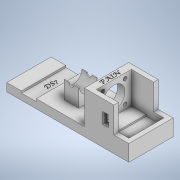
# Autodesk Inventor part: GN_StepperMount_v3
Saved by Autodesk Inventor 2020 (Build 240168000, 168)
## iProperties
Created: 2021-12-03
Part Number: GN_StepperMount_v3
Material: Generic
Document SubType Name: Modeling
Designer: bi19884
Density: 1 g/cm^3
Appearance: Default
Author: bi19884
Autodesk Inventor part; units mm, degrees
ref_plane "YZ Plane" through (0, 0, 0) normal (1, 0, 0) x (0, 1, 0)
ref_plane "XZ Plane" through (0, 0, 0) normal (0, 1, 0) x (-1, 0, 0)
ref_plane "XY Plane" through (0, 0, 0) normal (0, 0, 1) x (1, 0, 0)
sketch "Sketch1" plane through (0, 0, 0) normal (0, 1, 0) x (-1, 0, 0)
  line L0 (10.1329, 50.4274) -> (-115.1171, 50.4274)
  line L1 (-115.1171, 50.4274) -> (-115.1171, -9.5726)
  line L2 (-115.1171, -9.5726) -> (10.1329, -9.5726)
  line L3 (10.1329, -9.5726) -> (10.1329, 50.4274)
  point P0 (0, 0)
  dimension "d0" = 125.25
  dimension "d1" = 60
  constraints: 8 end point, 2 parallel, 1 horizontal, 1 perpendicular
  measures "d0" distance of L1.end L2.end
  measures "d1" distance of L2.end L0.start
extrude "Extrusion1" add sketch "Sketch1" along normal blind 12
sketch "Sketch2" plane through (-10.1329, 0, -9.5726) normal (-1, 0, 0) x (0, 0, 1)
  line L0 (0, 8.5) -> (60, 8.5)
  line L1 (60, 8.5) -> (60, 0)
  line L2 (60, 0) -> (0, 0)
  line L3 (0, 0) -> (0, 8.5)
  line L4 (0, 0) -> (0, 12) projected
  line L5 (0, 0) -> (60, 0) projected
  point P0 (9.5726, 0)
  dimension "d4" = 8.5
  dimension "d5" = 60
  dimension "d6" = 0
  dimension "d7" = 0
  constraints: 8 end point, 2 parallel, 1 horizontal, 1 perpendicular
  measures "d4" distance between parallel lines of L0 L2
  measures "d5" distance between parallel lines of L1 L3
  measures "d6" distance between parallel lines of L4 L3
  measures "d7" distance between parallel lines of L5 L2
extrude "Extrusion2" add sketch "Sketch2" along normal blind 40
sketch "Sketch4" plane through (0, 12, 0) normal (0, 1, 0) x (1, 0, 0)
  line L0 (115.1171, 9.5726) -> (-10.1329, 9.5726) projected
  line L1 (-10.1329, -50.4274) -> (115.1171, -50.4274) projected
  line L2 (115.1171, -50.4274) -> (115.1171, 9.5726) projected
  line L3 (-10.1329, 9.5726) -> (-10.1329, -50.4274) projected
  line L4 (9.8671, -7.9274) -> (29.8671, -7.9274)
  line L5 (29.8671, -7.9274) -> (29.8671, -32.9274)
  line L6 (29.8671, -32.9274) -> (9.8671, -32.9274)
  line L7 (9.8671, -32.9274) -> (9.8671, -7.9274)
  point P0 (0, 0)
  dimension "d15" = 60
  dimension "d16" = 125.25
  dimension "d17" = 25
  dimension "d18" = 20
  dimension "d19" = 17.5
  dimension "d20" = 17.5
  dimension "d21" = 20
  constraints: 8 end point, 2 parallel, 1 horizontal, 1 perpendicular
  measures "d15" distance between parallel lines of L0 L1
  measures "d16" distance between parallel lines of L2 L3
  measures "d17" distance between parallel lines of L4 L6
  measures "d18" distance between parallel lines of L5 L7
  measures "d19" distance between parallel lines of L1 L6
  measures "d20" distance between parallel lines of L0 L4
  measures "d21" distance between parallel lines of L3 L7
extrude "Extrusion3" add sketch "Sketch4" along normal blind 23.5 contours L4 L5 L6 L7
sketch "Sketch6" plane through (29.8671, 12, 32.9274) normal (1, 0, 0) x (0, 0, -1)
  circle A0 centre (12.5, 23.5) radius 11.5
  line L0 (0, 23.5) -> (25, 23.5) projected
  line L1 (25, 0) -> (25, 23.5) projected
  line L2 (0, 0) -> (0, 23.5) projected
  line L3 (-17.5, 0) -> (42.5, 0) projected
  point P0 (32.9274, -12)
  point P1 (24, 23.5)
  point P2 (1, 23.5)
  dimension "d24" = 23
  dimension "d25" = 0
  dimension "d26" = 12.5
  dimension "d27" = 25
  dimension "d153" = 23.5
  constraints: 1 centre point
  measures "d24" diameter of A0
  measures "d25" distance from line of L0 A0.centre
  measures "d26" distance from line of L1 A0.centre
  measures "d27" distance between parallel lines of L2 L1
  measures "d153" distance from line of L3 A0.centre
extrude "Extrusion4" cut sketch "Sketch6" against normal blind 20 contours A0 L0 picked at (10.3224, 16.7824)
sketch "Sketch7" plane through (9.8671, 12, 32.9274) normal (0, 0, 1) x (1, 0, 0)
  circle A0 centre (10, 23.5) radius 3.5
  line L0 (0, 23.5) -> (20, 23.5) projected
  line L1 (0, 0) -> (0, 23.5) projected
  line L2 (20, 0) -> (20, 23.5) projected
  point P0 (-9.8671, -12)
  point P1 (13.5, 23.5)
  point P2 (6.5, 23.5)
  dimension "d30" = 7
  dimension "d31" = 0
  dimension "d32" = 20
  dimension "d33" = 10
  dimension "d34" = 10
  constraints: 1 centre point
  measures "d30" diameter of A0
  measures "d31" distance from line of L0 A0.centre
  measures "d32" distance between parallel lines of L1 L2
  measures "d33" distance from line of L2 A0.centre
  measures "d34" distance from line of L1 A0.centre
extrude "Extrusion5" cut sketch "Sketch7" against normal blind 25 contours A0 L0 picked at (11.1667, 22.4156)
sketch "Sketch8" plane through (0, 12, 0) normal (0, 1, 0) x (1, 0, 0)
  line L0 (64.8671, 9.5726) -> (54.8671, 9.5726)
  line L1 (54.8671, 9.5726) -> (54.8671, -50.4274)
  line L2 (54.8671, -50.4274) -> (64.8671, -50.4274)
  line L3 (64.8671, -50.4274) -> (64.8671, 9.5726)
  line L4 (-10.1329, 9.5726) -> (-10.1329, -50.4274) projected
  line L5 (-10.1329, -50.4274) -> (115.1171, -50.4274) projected
  line L6 (115.1171, 9.5726) -> (-10.1329, 9.5726) projected
  point P0 (0, 0)
  dimension "d37" = 65
  dimension "d38" = 10
  dimension "d39" = 0
  dimension "d40" = 60
  dimension "d41" = 60
  dimension "d42" = 0
  constraints: 8 end point, 2 parallel, 1 horizontal, 1 perpendicular
  measures "d37" distance between parallel lines of L4 L1
  measures "d38" distance between parallel lines of L1 L3
  measures "d39" distance between parallel lines of L5 L2
  measures "d40" distance of L0.end L1.end
  measures "d41" distance between parallel lines of L5 L6
  measures "d42" distance between parallel lines of L6 L0
extrude "Extrusion6" add sketch "Sketch8" along normal blind 45 contours L3 L2 L1 L0
sketch "Sketch9" plane through (0, 12, 0) normal (0, 1, 0) x (1, 0, 0)
  line L0 (108.8671, 9.5726) -> (115.1171, 9.5726)
  line L1 (115.1171, 9.5726) -> (115.1171, -50.4274)
  line L2 (115.1171, -50.4274) -> (108.8671, -50.4274)
  line L3 (108.8671, -50.4274) -> (108.8671, 9.5726)
  line L4 (64.8671, -50.4274) -> (64.8671, 9.5726) projected
  line L5 (54.8671, 9.5726) -> (54.8671, -50.4274) projected
  line L6 (29.8671, -8.9274) -> (29.8671, -31.9274) projected
  line L7 (115.1171, 9.5726) -> (-10.1329, 9.5726) projected
  line L8 (64.8671, 9.5726) -> (54.8671, 9.5726) projected
  line L9 (-10.1329, -50.4274) -> (115.1171, -50.4274) projected
  line L10 (54.8671, -50.4274) -> (64.8671, -50.4274) projected
  line L11 (115.1171, -50.4274) -> (115.1171, 9.5726) projected
  point P0 (0, 0)
  dimension "d45" = 6.25
  dimension "d46" = 44
  dimension "d47" = 25
  dimension "d48" = 0
  dimension "d49" = 60
  dimension "d50" = 0
  dimension "d51" = 0
  dimension "d52" = 60
  dimension "d69" = 0
  constraints: 8 end point, 2 parallel, 1 horizontal, 1 perpendicular
  measures "d45" distance between parallel lines of L1 L3
  measures "d46" distance between parallel lines of L4 L3
  measures "d47" distance between parallel lines of L5 L6
  measures "d48" distance between parallel lines of L7 L0
  measures "d49" distance between parallel lines of L2 L0
  measures "d50" distance between parallel lines of L7 L8
  measures "d51" distance from line of L9 L2.end
  measures "d52" distance between parallel lines of L10 L8
  measures "d69" distance between parallel lines of L11 L1
extrude "Extrusion7" add sketch "Sketch9" along normal blind 10 contours L0 L1 L2 L3
sketch "Sketch10" plane through (64.8671, 12, 50.4274) normal (1, 0, 0) x (0, 0, -1)
  circle A0 centre (30, 23.5) radius 15
  line L0 (0, 0) -> (0, 45) projected
  line L1 (60, 0) -> (60, 45) projected
  line L2 (0, 0) -> (60, 0) projected
  line L3 (0, 45) -> (60, 45) projected
  point P0 (50.4274, -12)
  dimension "d55" = 30
  dimension "d56" = 30
  dimension "d57" = 30
  dimension "d58" = 60
  dimension "d59" = 23.5
  dimension "d60" = 21.5
  constraints: 1 centre point
  measures "d55" diameter of A0
  measures "d56" distance from line of L0 A0.centre
  measures "d57" distance from line of L1 A0.centre
  measures "d58" distance between parallel lines of L1 L0
  measures "d59" distance from line of L2 A0.centre
  measures "d60" distance from line of L3 A0.centre
extrude "Extrusion8" cut sketch "Sketch10" against normal blind 10 contours A0
sketch "Sketch12" plane through (0, 12, 0) normal (0, 1, 0) x (1, 0, 0)
  line L0 (64.8671, 3.3226) -> (84.8671, 3.3226)
  line L1 (84.8671, 3.3226) -> (84.8671, -44.1774)
  line L2 (84.8671, -44.1774) -> (64.8671, -44.1774)
  line L3 (64.8671, -44.1774) -> (64.8671, 3.3226)
  line L4 (64.8671, -50.4274) -> (64.8671, 9.5726) projected
  line L5 (54.8671, -50.4274) -> (64.8671, -50.4274) projected
  line L6 (108.8671, 9.5726) -> (64.8671, 9.5726) projected
  line L7 (64.8671, -50.4274) -> (108.8671, -50.4274) projected
  point P0 (0, 0)
  dimension "d63" = 20
  dimension "d64" = 47.5
  dimension "d65" = 0
  dimension "d132" = 6.25
  dimension "d133" = 6.25
  constraints: 8 end point, 2 parallel, 1 horizontal, 1 perpendicular
  measures "d63" distance of L0.start L0.end
  measures "d64" distance of L0.end L1.end
  measures "d65" distance between parallel lines of L4 L3
  measures "d132" distance between parallel lines of L0 L6
  measures "d133" distance between parallel lines of L7 L2
extrude "Extrusion9" add sketch "Sketch12" along normal blind 2
sketch "Sketch13" plane through (64.8671, 57, 50.4274) normal (1, 0, 0) x (0, 0, -1)
  circle A0 centre (15, -6.5) radius 2.5
  line L0 (0, 0) -> (60, 0) projected
  line L1 (0, -43) -> (0, 0) projected
  circle A1 centre (45, -6.5) radius 2.5
  line L2 (60, -43) -> (60, 0) projected
  circle A2 centre (15, -36.5) radius 2.5
  circle A3 centre (45, -36.5) radius 2.5
  circle A4 centre (30, -21.5) radius 15 projected
  line L3 (6.25, -43) -> (53.75, -43) projected
  point P0 (50.4274, -57)
  dimension "d70" = 5
  dimension "d71" = 6.5
  dimension "d72" = 15
  dimension "d73" = 5
  dimension "d74" = 6.5
  dimension "d75" = 15
  dimension "d76" = 30
  dimension "d77" = 5
  dimension "d78" = 30
  dimension "d79" = 30
  dimension "d80" = 0
  dimension "d81" = 0
  dimension "d84" = 15
  dimension "d85" = 15
  dimension "d111" = 6.5
  constraints: 4 centre point
  measures "d70" diameter of A0
  measures "d71" distance from line of L0 A0.centre
  measures "d72" distance from line of L1 A0.centre
  measures "d73" diameter of A1
  measures "d74" distance from line of L0 A1.centre
  measures "d75" distance from line of L2 A1.centre
  measures "d76" distance of A1.centre A0.centre
  measures "d77" diameter of A2
  measures "d78" distance of A1.centre A3.centre
  measures "d79" distance of A0.centre A2.centre
  measures "d80" horizontal distance of A2.centre A0.centre
  measures "d81" horizontal distance of A1.centre A3.centre
  measures "d84" horizontal distance of A4.centre A1.centre
  measures "d85" horizontal distance of A2.centre A4.centre
  measures "d111" distance from line of A2.centre L3
extrude "Extrusion10" cut sketch "Sketch13" against normal blind 10 contours A0 | A1 | A2 | A3
sketch "Sketch14" plane through (0, 57, 0) normal (0, 1, 0) x (1, 0, 0)
  line L0 (54.8671, -35.4274) -> (54.8671, -5.4274) construction
  line L1 (54.8671, -5.4274) -> (64.8671, -5.4274) construction
  line L2 (64.8671, -5.4274) -> (64.8671, -35.4274) construction
  line L3 (64.8671, -35.4274) -> (54.8671, -35.4274) construction
  line L4 (-10.1329, -50.4274) -> (115.1171, -50.4274) projected
  line L5 (115.1171, 9.5726) -> (-10.1329, 9.5726) projected
  line L6 (54.8671, 9.5726) -> (54.8671, -50.4274) projected
  line L7 (62.7624, -33.3703) -> (62.1814, -32.7844)
  line L8 (62.1814, -32.7844) -> (62.1814, -32.7105)
  line L9 (62.1814, -32.7105) -> (62.1863, -32.5431)
  spline S0 degree 2 poles (62.1863, -32.5431) (62.1863, -32.0753) (61.5708, -31.6518) (60.6303, -31.4647) knots 0 0 0 1 2 2 2
  line L10 (60.6303, -31.4647) -> (57.2622, -30.795)
  spline S1 degree 2 poles (57.2622, -30.795) (57.2622, -31.6026) (58.1289, -32.6022) (58.8281, -32.6022) knots 0 0 0 1 2 2 2
  line L11 (58.8281, -32.6022) -> (58.9118, -32.6022)
  line L12 (58.9118, -32.6022) -> (59.2811, -33.3654)
  spline S2 degree 2 poles (59.2811, -33.3654) (58.0599, -33.2571) (56.9471, -31.5829) (56.9471, -29.8447) knots 0 0 0 1 2 2 2
  spline S3 degree 2 poles (56.9471, -29.8447) (56.9471, -28.594) (57.4838, -27.5304) (58.1141, -27.5304) knots 0 0 0 1 2 2 2
  spline S4 degree 2 poles (58.1141, -27.5304) (58.6164, -27.5304) (59.6603, -28.2592) (59.9459, -28.8156) knots 0 0 0 1 2 2 2
  spline S5 degree 2 poles (59.9459, -28.8156) (60.2659, -29.4557) (60.2659, -30.278) knots 0 0 0 1 1 1
  line L13 (60.2659, -30.278) -> (60.2659, -30.3814)
  line L14 (60.2659, -30.3814) -> (60.0246, -30.2337)
  line L15 (60.0246, -30.2337) -> (60.0246, -30.1648)
  spline S6 degree 2 poles (60.0246, -30.1648) (60.0246, -29.4065) (59.0349, -28.3872) (58.2963, -28.3872) knots 0 0 0 1 2 2 2
  spline S7 degree 2 poles (58.2963, -28.3872) (57.1884, -28.3872) (57.1884, -29.958) knots 0 0 0 1 1 1
  line L16 (57.1884, -29.958) -> (60.3693, -30.5932)
  spline S8 degree 2 poles (60.3693, -30.5932) (61.5708, -30.8295) (62.2503, -31.8931) knots 0 0 0 1 1 1
  line L17 (62.2503, -31.8931) -> (62.2799, -30.3814)
  line L18 (62.2799, -30.3814) -> (62.8609, -30.9231)
  line L19 (62.8609, -30.9231) -> (62.7624, -33.3703)
  line L20 (62.4276, -27.683) -> (61.8909, -27.1512)
  spline S9 degree 2 poles (61.8909, -27.1512) (62.467, -26.777) (62.467, -26.1713) knots 0 0 0 1 1 1
  spline S10 degree 2 poles (62.467, -26.1713) (62.467, -25.5952) (61.5068, -24.5809) (60.2807, -23.8718) knots 0 0 0 1 2 2 2
  line L21 (60.2807, -23.8718) -> (57.3558, -22.1779)
  spline S11 degree 2 poles (57.3558, -22.1779) (57.3066, -22.6063) (57.3066, -22.9116) knots 0 0 0 1 1 1
  spline S12 degree 2 poles (57.3066, -22.9116) (57.3066, -23.7339) (58.1289, -24.6252) (58.8921, -24.6252) knots 0 0 0 1 2 2 2
  line L22 (58.8921, -24.6252) -> (59.2713, -25.3983)
  spline S13 degree 2 poles (59.2713, -25.3983) (58.5326, -25.3244) (58.0501, -24.9846) knots 0 0 0 1 1 1
  spline S14 degree 2 poles (58.0501, -24.9846) (57.5134, -24.6104) (57.0554, -23.5961) (56.9865, -22.6359) knots 0 0 0 1 2 2 2
  spline S15 degree 2 poles (56.9865, -22.6359) (56.9766, -22.4438) (56.9471, -22.0548) knots 0 0 0 1 1 1
  line L23 (56.9471, -22.0548) -> (56.7994, -21.2522)
  line L24 (56.7994, -21.2522) -> (58.1092, -21.203)
  line L25 (58.1092, -21.203) -> (60.8223, -20.9715)
  spline S16 degree 2 poles (60.8223, -20.9715) (61.7678, -20.8927) (62.3685, -20.6071) (62.3685, -20.2329) knots 0 0 0 1 2 2 2
  spline S17 degree 2 poles (62.3685, -20.2329) (62.3685, -20.1689) (62.3439, -19.775) knots 0 0 0 1 1 1
  line L26 (62.3439, -19.775) -> (62.6049, -19.8242)
  line L27 (62.6049, -19.8242) -> (62.9052, -21.6314)
  line L28 (62.9052, -21.6314) -> (60.9701, -21.7889)
  line L29 (60.9701, -21.7889) -> (60.9701, -23.9309)
  spline S18 degree 2 poles (60.9701, -23.9309) (62.0435, -24.5513) (62.9052, -25.6592) (62.9052, -26.4274) knots 0 0 0 1 2 2 2
  spline S19 degree 2 poles (62.9052, -26.4274) (62.9052, -27.1512) (62.4276, -27.683) knots 0 0 0 1 1 1
  line L30 (60.6795, -23.7635) -> (60.6795, -21.8185)
  line L31 (60.6795, -21.8185) -> (57.7251, -22.0696)
  line L32 (57.7251, -22.0696) -> (60.6795, -23.7635)
  line L33 (62.7624, -20.1492) -> (62.1814, -19.5583)
  line L34 (62.1814, -19.5583) -> (62.1814, -19.2973)
  spline S20 degree 2 poles (62.1814, -19.2973) (62.1814, -18.8493) (61.5954, -18.4209) (60.7337, -18.2534) knots 0 0 0 1 2 2 2
  line L35 (60.7337, -18.2534) -> (57.5281, -17.6133)
  line L36 (57.5281, -17.6133) -> (57.5281, -18.6769)
  line L37 (57.5281, -18.6769) -> (56.9471, -18.1057)
  line L38 (56.9471, -18.1057) -> (56.9471, -15.5501)
  line L39 (56.9471, -15.5501) -> (57.5281, -16.1459)
  line L40 (57.5281, -16.1459) -> (57.5281, -16.7861)
  line L41 (57.5281, -16.7861) -> (60.3102, -17.3425)
  spline S21 degree 2 poles (60.3102, -17.3425) (61.5856, -17.5985) (62.2405, -18.6621) knots 0 0 0 1 1 1
  line L42 (62.2405, -18.6621) -> (62.2799, -17.1308)
  line L43 (62.2799, -17.1308) -> (62.8609, -17.697)
  line L44 (62.8609, -17.697) -> (62.7624, -20.1492)
  line L45 (62.3931, -16.2493) -> (61.8219, -15.688)
  spline S22 degree 2 poles (61.8219, -15.688) (62.4719, -15.2891) (62.4719, -14.5899) knots 0 0 0 1 1 1
  spline S23 degree 2 poles (62.4719, -14.5899) (62.4719, -14.1221) (61.689, -13.4032) (61.039, -13.2752) knots 0 0 0 1 2 2 2
  line L46 (61.039, -13.2752) -> (57.3066, -12.5317)
  spline S24 degree 2 poles (57.3066, -12.5317) (57.277, -12.7336) (57.277, -12.8173) knots 0 0 0 1 1 1
  spline S25 degree 2 poles (57.277, -12.8173) (57.277, -13.4623) (58.2027, -14.324) (58.8872, -14.324) knots 0 0 0 1 2 2 2
  line L47 (58.8872, -14.324) -> (59.2614, -15.0873)
  spline S26 degree 2 poles (59.2614, -15.0873) (58.2224, -15.0085) (56.9471, -13.4623) (56.9471, -12.2756) knots 0 0 0 1 2 2 2
  line L48 (56.9471, -12.2756) -> (56.9471, -11.8965)
  spline S27 degree 2 poles (56.9471, -11.8965) (57.9861, -11.4927) (59.158, -10.8329) knots 0 0 0 1 1 1
  line L49 (59.158, -10.8329) -> (60.0493, -10.3355)
  spline S28 degree 2 poles (60.0493, -10.3355) (60.9651, -9.8087) (61.5265, -9.5674) knots 0 0 0 1 1 1
  line L50 (61.5265, -9.5674) -> (59.2565, -9.1144)
  spline S29 degree 2 poles (59.2565, -9.1144) (58.0846, -8.8829) (56.7994, -7.7307) (56.7994, -6.9133) knots 0 0 0 1 2 2 2
  spline S30 degree 2 poles (56.7994, -6.9133) (56.7994, -6.6228) (56.9077, -6.3421) knots 0 0 0 1 1 1
  line L51 (56.9077, -6.3421) -> (57.4395, -6.6228)
  spline S31 degree 2 poles (57.4395, -6.6228) (57.1638, -6.9724) (57.1638, -7.2974) knots 0 0 0 1 1 1
  spline S32 degree 2 poles (57.1638, -7.2974) (57.1638, -8.1443) (58.641, -8.4348) knots 0 0 0 1 1 1
  line L52 (58.641, -8.4348) -> (61.6003, -9.0257)
  line L53 (61.6003, -9.0257) -> (62.7624, -9.2079)
  line L54 (62.7624, -9.2079) -> (62.9348, -9.7102)
  spline S33 degree 2 poles (62.9348, -9.7102) (62.4916, -9.853) (61.2754, -10.5374) knots 0 0 0 1 1 1
  line L55 (61.2754, -10.5374) -> (59.5716, -11.4976)
  spline S34 degree 2 poles (59.5716, -11.4976) (58.8872, -11.8866) (58.3505, -12.1377) knots 0 0 0 1 1 1
  line L56 (58.3505, -12.1377) -> (59.8621, -12.4332)
  spline S35 degree 2 poles (59.8621, -12.4332) (61.2951, -12.7237) (62.8363, -14.0631) (62.8363, -15.0232) knots 0 0 0 1 2 2 2
  spline S36 degree 2 poles (62.8363, -15.0232) (62.8363, -15.6978) (62.3931, -16.2493) knots 0 0 0 1 1 1
  point P0 (0, 0)
  dimension "d86" = 30
  dimension "d87" = 10
  dimension "d88" = 15
  dimension "d89" = 15
  dimension "d90" = 0
  constraints: 2 other
  measures "d86" distance between parallel lines of L1 L3
  measures "d87" distance of L0.end L1.end
  measures "d88" distance between parallel lines of L4 L3
  measures "d89" distance between parallel lines of L5 L1
  measures "d90" distance between parallel lines of L6 L0
extrude "Extrusion12" cut sketch "Sketch14" against normal blind 0.5
sketch "Sketch15" plane through (-10.1329, 8.5, 50.4274) normal (0, 1, 0) x (1, 0, 0)
  line L0 (-15, 20) -> (-15, 40) construction
  line L1 (-15, 40) -> (-5, 40) construction
  line L2 (-5, 40) -> (-5, 20) construction
  line L3 (-5, 20) -> (-15, 20) construction
  line L4 (0, 0) -> (-40, 0) projected
  line L5 (0, 60) -> (-40, 60) projected
  line L6 (-40, 0) -> (-40, 60) projected
  line L7 (0, 60) -> (0, 0) projected
  line L8 (-7.6488, 22.3086) -> (-8.2298, 22.8847)
  line L9 (-8.2298, 22.8847) -> (-8.2396, 22.9438)
  spline S0 degree 2 poles (-8.2396, 22.9438) (-8.2396, 22.9684) (-8.2347, 23.0472) knots 0 0 0 1 1 1
  spline S1 degree 2 poles (-8.2347, 23.0472) (-8.2298, 23.0866) (-8.2298, 23.1309) knots 0 0 0 1 1 1
  spline S2 degree 2 poles (-8.2298, 23.1309) (-8.2298, 23.5593) (-8.7517, 23.9976) (-9.4263, 24.1305) knots 0 0 0 1 2 2 2
  line L10 (-9.4263, 24.1305) -> (-13.1588, 24.874)
  spline S3 degree 2 poles (-13.1588, 24.874) (-13.1588, 24.0665) (-12.2922, 23.0669) (-11.5929, 23.0669) knots 0 0 0 1 2 2 2
  line L11 (-11.5929, 23.0669) -> (-11.5043, 23.0669)
  line L12 (-11.5043, 23.0669) -> (-11.135, 22.3037)
  spline S4 degree 2 poles (-11.135, 22.3037) (-13.4641, 22.5105) (-13.4641, 25.6619) knots 0 0 0 1 1 1
  line L13 (-13.4641, 25.6619) -> (-13.4641, 26.7944)
  spline S5 degree 2 poles (-13.4641, 26.7944) (-13.4641, 28.1092) (-12.4842, 29.2712) (-11.3763, 29.2712) knots 0 0 0 1 2 2 2
  spline S6 degree 2 poles (-11.3763, 29.2712) (-9.5839, 29.2712) (-7.5503, 26.7895) (-7.5503, 24.6081) knots 0 0 0 1 2 2 2
  spline S7 degree 2 poles (-7.5503, 24.6081) (-7.5503, 24.5146) (-7.5601, 24.2388) knots 0 0 0 1 1 1
  line L14 (-7.5601, 24.2388) -> (-7.6488, 22.3086)
  line L15 (-8.1461, 23.7267) -> (-8.0279, 24.426)
  spline S8 degree 2 poles (-8.0279, 24.426) (-7.9294, 24.9971) (-7.9294, 25.588) knots 0 0 0 1 1 1
  spline S9 degree 2 poles (-7.9294, 25.588) (-7.9294, 26.3956) (-8.3726, 27.3016) (-8.9635, 27.6857) knots 0 0 0 1 2 2 2
  spline S10 degree 2 poles (-8.9635, 27.6857) (-9.9975, 28.3652) (-11.2679, 28.3652) knots 0 0 0 1 1 1
  spline S11 degree 2 poles (-11.2679, 28.3652) (-13.2228, 28.3652) (-13.2228, 26.2035) knots 0 0 0 1 1 1
  line L16 (-13.2228, 26.2035) -> (-13.2228, 25.7111)
  line L17 (-13.2228, 25.7111) -> (-10.2093, 25.1104)
  spline S12 degree 2 poles (-10.2093, 25.1104) (-9.387, 24.9479) (-8.5499, 24.3816) (-8.1461, 23.7267) knots 0 0 0 1 2 2 2
  line L18 (-7.8703, 29.7587) -> (-8.4268, 30.3053)
  spline S13 degree 2 poles (-8.4268, 30.3053) (-7.8457, 31.0291) (-7.8457, 31.8071) knots 0 0 0 1 1 1
  spline S14 degree 2 poles (-7.8457, 31.8071) (-7.8457, 32.3439) (-8.4514, 33.0283) (-8.9339, 33.0283) knots 0 0 0 1 2 2 2
  spline S15 degree 2 poles (-8.9339, 33.0283) (-9.4017, 33.0283) (-9.9729, 32.3833) knots 0 0 0 1 1 1
  line L19 (-9.9729, 32.3833) -> (-10.4604, 31.8268)
  spline S16 degree 2 poles (-10.4604, 31.8268) (-11.007, 31.2113) (-11.4452, 30.9159) (-11.8145, 30.9159) knots 0 0 0 1 2 2 2
  spline S17 degree 2 poles (-11.8145, 30.9159) (-12.5482, 30.9159) (-13.6118, 32.1567) (-13.6118, 33.0185) knots 0 0 0 1 2 2 2
  spline S18 degree 2 poles (-13.6118, 33.0185) (-13.6118, 33.565) (-13.2868, 34.2987) knots 0 0 0 1 1 1
  line L20 (-13.2868, 34.2987) -> (-12.302, 34.1018)
  line L21 (-12.302, 34.1018) -> (-12.302, 33.8555)
  spline S19 degree 2 poles (-12.302, 33.8555) (-12.4251, 33.8654) (-12.4694, 33.8654) knots 0 0 0 1 1 1
  spline S20 degree 2 poles (-12.4694, 33.8654) (-12.8437, 33.8654) (-13.2967, 33.2647) (-13.2967, 32.7723) knots 0 0 0 1 2 2 2
  spline S21 degree 2 poles (-13.2967, 32.7723) (-13.2967, 32.2651) (-12.6959, 31.5757) (-12.2528, 31.5757) knots 0 0 0 1 2 2 2
  spline S22 degree 2 poles (-12.2528, 31.5757) (-11.9524, 31.5757) (-11.46, 31.9253) (-10.9873, 32.4817) knots 0 0 0 1 2 2 2
  line L22 (-10.9873, 32.4817) -> (-10.5884, 32.9446)
  spline S23 degree 2 poles (-10.5884, 32.9446) (-9.9237, 33.7177) (-9.3476, 33.7177) knots 0 0 0 1 1 1
  spline S24 degree 2 poles (-9.3476, 33.7177) (-8.5893, 33.7177) (-7.506, 32.2651) (-7.506, 31.2556) knots 0 0 0 1 2 2 2
  spline S25 degree 2 poles (-7.506, 31.2556) (-7.506, 30.4875) (-7.8703, 29.7587) knots 0 0 0 1 1 1
  spline S26 degree 2 poles (-6.3882, 34.5006) (-7.2499, 34.6582) (-8.1855, 35.4608) knots 0 0 0 1 1 1
  line L23 (-8.1855, 35.4608) -> (-10.7608, 37.8884)
  line L24 (-10.7608, 37.8884) -> (-11.2335, 38.3118)
  line L25 (-11.2335, 38.3118) -> (-11.2335, 35.0767)
  line L26 (-11.2335, 35.0767) -> (-11.913, 35.3525)
  line L27 (-11.913, 35.3525) -> (-11.913, 39.0504)
  line L28 (-11.913, 39.0504) -> (-11.4748, 38.8732)
  spline S27 degree 2 poles (-11.4748, 38.8732) (-8.0328, 35.643) (-6.4867, 35.4263) knots 0 0 0 1 1 1
  line L29 (-6.4867, 35.4263) -> (-6.3882, 34.5006)
  point P0 (10.1329, 50.4274)
  dimension "d95" = 20
  dimension "d96" = 20
  dimension "d97" = 20
  dimension "d98" = 25
  dimension "d99" = 10
  dimension "d100" = 40
  constraints: 2 other
  measures "d95" distance between parallel lines of L4 L3
  measures "d96" distance of L0.start L0.end
  measures "d97" distance between parallel lines of L5 L1
  measures "d98" distance between parallel lines of L6 L0
  measures "d99" distance of L0.end L1.end
  measures "d100" distance between parallel lines of L6 L7
extrude "Extrusion13" cut sketch "Sketch15" against normal blind 0.5 contours L8 L9 S0 S1 S2 L10 S3 L11 L12 S4 L13 S5 S6 S7 L14 | L18 S13 S14 S15 L19 S16 S17 S18 L20 L21 S19 S20 S21 S22 L22 S23 S24 S25 | S26 L23 L24 L25 L26 L27 L28 S27 L29
sketch "Sketch21" plane through (0, 12, 0) normal (0, 1, 0) x (1, 0, 0)
  line L0 (64.8671, 9.5726) -> (108.8671, 9.5726)
  line L1 (108.8671, 9.5726) -> (108.8671, 3.3226)
  line L2 (108.8671, 3.3226) -> (64.8671, 3.3226)
  line L3 (64.8671, 3.3226) -> (64.8671, 9.5726)
  line L4 (108.8671, 9.5726) -> (108.8671, -50.4274) projected
  line L5 (64.8671, -50.4274) -> (64.8671, 9.5726) projected
  line L6 (108.8671, 9.5726) -> (64.8671, 9.5726) projected
  line L7 (64.8671, -44.1774) -> (108.8671, -44.1774)
  line L8 (108.8671, -44.1774) -> (108.8671, -50.4274)
  line L9 (108.8671, -50.4274) -> (64.8671, -50.4274)
  line L10 (64.8671, -50.4274) -> (64.8671, -44.1774)
  line L11 (64.8671, -50.4274) -> (108.8671, -50.4274) projected
  point P0 (0, 0)
  dimension "d134" = 44
  dimension "d135" = 44
  dimension "d136" = 0
  dimension "d137" = 0
  dimension "d138" = 44
  dimension "d139" = 6.25
  dimension "d140" = 0
  dimension "d141" = 0
  dimension "d142" = 47.5
  dimension "d143" = 6.25
  constraints: 16 end point, 4 parallel, 2 horizontal, 2 perpendicular
  measures "d134" distance between parallel lines of L4 L5
  measures "d135" distance between parallel lines of L1 L3
  measures "d136" distance between parallel lines of L5 L3
  measures "d137" distance between parallel lines of L6 L0
  measures "d138" distance of L8.end L9.end
  measures "d139" distance of L0.end L1.end
  measures "d140" distance between parallel lines of L5 L10
  measures "d141" distance between parallel lines of L11 L9
  measures "d142" distance between parallel lines of L7 L2
  measures "d143" distance between parallel lines of L9 L7
extrude "Extrusion15" add sketch "Sketch21" along normal blind 10 contours L0 L1 L2 L3 | L7 L4 L9 L5
sketch "Sketch22" plane through (-10.1329, 8.5, 50.4274) normal (0, 1, 0) x (1, 0, 0)
  line L0 (-40, 60) -> (-20, 60)
  line L1 (-20, 60) -> (-20, 0)
  line L2 (-20, 0) -> (-40, 0)
  line L3 (-40, 0) -> (-40, 60)
  line L4 (0, 60) -> (-40, 60) projected
  line L5 (0, 60) -> (0, 0) projected
  line L6 (-40, 0) -> (-40, 60) projected
  point P0 (10.1329, 50.4274)
  dimension "d146" = 20
  dimension "d147" = 60
  dimension "d148" = 0
  dimension "d150" = 0
  constraints: 8 end point, 2 parallel, 1 horizontal, 1 perpendicular
  measures "d146" distance of L0.start L0.end
  measures "d147" distance of L2.end L0.start
  measures "d148" distance between parallel lines of L4 L0
  measures "d150" distance between parallel lines of L6 L3
extrude "Extrusion16" add sketch "Sketch22" along normal blind 2.5
sketch "Sketch23" plane through (0, 22, 0) normal (0, 1, 0) x (1, 0, 0)
  line L0 (64.8671, 3.3226) -> (94.8671, 3.3226)
  line L1 (94.8671, 3.3226) -> (94.8671, 9.5726)
  line L2 (94.8671, 9.5726) -> (64.8671, 9.5726)
  line L3 (64.8671, 9.5726) -> (64.8671, 3.3226)
  line L4 (115.1171, 9.5726) -> (64.8671, 9.5726) projected
  line L5 (64.8671, 3.3226) -> (108.8671, 3.3226) projected
  line L6 (64.8671, -50.4274) -> (64.8671, 9.5726) projected
  line L7 (64.8671, -44.1774) -> (94.8671, -44.1774)
  line L8 (94.8671, -44.1774) -> (94.8671, -50.4274)
  line L9 (94.8671, -50.4274) -> (64.8671, -50.4274)
  line L10 (64.8671, -50.4274) -> (64.8671, -44.1774)
  line L11 (108.8671, -44.1774) -> (64.8671, -44.1774) projected
  point P0 (0, 0)
  dimension "d154" = 30
  dimension "d155" = 6.25
  dimension "d156" = 6.25
  dimension "d157" = 0
  dimension "d158" = 0
  dimension "d159" = 30
  dimension "d160" = 6.25
  dimension "d161" = 0
  dimension "d162" = 0
  constraints: 16 end point, 4 parallel, 2 horizontal, 2 perpendicular
  measures "d154" distance of L1.end L2.end
  measures "d155" distance between parallel lines of L4 L5
  measures "d156" distance between parallel lines of L2 L0
  measures "d157" distance between parallel lines of L6 L3
  measures "d158" distance between parallel lines of L5 L0
  measures "d159" distance of L8.end L9.end
  measures "d160" distance of L7.end L8.end
  measures "d161" distance between parallel lines of L6 L10
  measures "d162" distance between parallel lines of L11 L7
extrude "Extrusion17" add sketch "Sketch23" along normal blind 35
sketch "Sketch24" plane through (-50.1329, 0, 50.4274) normal (0, 0, 1) x (1, 0, 0)
  line L0 (130, 42) -> (138, 42)
  line L1 (138, 42) -> (138, 27)
  line L2 (138, 27) -> (130, 27)
  line L3 (130, 27) -> (130, 42)
  line L4 (115, 57) -> (115, 14) projected
  line L5 (105, 12) -> (105, 57) projected
  line L6 (145, 22) -> (165.25, 22) projected
  line L7 (145, 22) -> (145, 57) projected
  line L8 (105, 57) -> (145, 57) projected
  point P0 (50.1329, 0)
  dimension "d165" = 10
  dimension "d166" = 15
  dimension "d167" = 15
  dimension "d168" = 8
  dimension "d169" = 5
  dimension "d170" = 7
  dimension "d171" = 15
  constraints: 8 end point, 2 parallel, 1 horizontal, 1 perpendicular
  measures "d165" distance between parallel lines of L4 L5
  measures "d166" distance between parallel lines of L3 L4
  measures "d167" distance of L2.end L0.start
  measures "d168" distance of L0.start L0.end
  measures "d169" distance between parallel lines of L2 L6
  measures "d170" distance between parallel lines of L7 L1
  measures "d171" distance between parallel lines of L8 L0
extrude "Extrusion18" cut sketch "Sketch24" against normal blind 6.25
body "Solid1"
